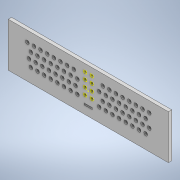
# Autodesk Inventor part: Front Panel
Saved by Autodesk Inventor 2021.4 (Build 254397000, 397)
## iProperties
Created: 2022-05-05
Part Number: Front Panel
Material: Generic
Document SubType Name: Modeling
Designer: LaborAdmin
Density: 1 g/cm^3
Appearance: Default
Author: LaborAdmin
Autodesk Inventor part; units mm, degrees
ref_plane "YZ Plane" through (0, 0, 0) normal (1, 0, 0) x (0, 1, 0)
ref_plane "XZ Plane" through (0, 0, 0) normal (0, 1, 0) x (-1, 0, 0)
ref_plane "XY Plane" through (0, 0, 0) normal (0, 0, 1) x (1, 0, 0)
sketch "Sketch1" plane through (0, 0, 0) normal (0, 0, 1) x (1, 0, 0)
  line L0 (241, -66.5) -> (-241, -66.5)
  line L1 (-241, -66.5) -> (-241, 66.5)
  line L2 (-241, 66.5) -> (241, 66.5)
  line L3 (241, 66.5) -> (241, -66.5)
  line L4 (241, -66.5) -> (-241, 66.5) construction
  line L5 (-241, -66.5) -> (241, 66.5) construction
  line L6 (197, -50) -> (-197, -50)
  line L7 (-197, -50) -> (-197, 50)
  line L8 (-197, 50) -> (197, 50)
  line L9 (197, 50) -> (197, -50)
  line L10 (197, -50) -> (-197, 50) construction
  line L11 (-197, -50) -> (197, 50) construction
  line L12 (25, 50) -> (25, -50) construction
  line L13 (-45, 50) -> (-45, -50) construction
  line L14 (-10, 45) -> (10, 45) construction
  line L15 (10, 45) -> (25, 45) construction
  line L16 (-10, 25) -> (-45, 25) construction
  line L17 (-10, 25) -> (10, 25) construction
  line L18 (-10, 5) -> (10, 5) construction
  line L19 (10, 5) -> (25, 5) construction
  arc A0 (-13.0692, 48.89) -> (-6.9308, 48.89) centre (-10, 45) ccw
  line L20 (-13.0692, 48.89) -> (-6.9308, 48.89)
  arc A1 (6.9308, 48.89) -> (13.0692, 48.89) centre (10, 45) ccw
  line L21 (6.9308, 48.89) -> (13.0692, 48.89)
  arc A2 (-13.0692, 28.89) -> (-6.9308, 28.89) centre (-10, 25) ccw
  arc A3 (6.9308, 28.89) -> (13.0692, 28.89) centre (10, 25) ccw
  arc A4 (6.9308, -11.11) -> (13.0692, -11.11) centre (10, -15) ccw
  arc A5 (-13.0692, -11.11) -> (-6.9308, -11.11) centre (-10, -15) ccw
  line L22 (-13.0692, 28.89) -> (-6.9308, 28.89)
  line L23 (6.9308, 28.89) -> (13.0692, 28.89)
  line L24 (-13.0692, -11.11) -> (-6.9308, -11.11)
  line L25 (6.9308, -11.11) -> (13.0692, -11.11)
  arc A6 (-13.0692, 8.89) -> (-6.9308, 8.89) centre (-10, 5) ccw
  arc A7 (6.9308, 8.89) -> (13.0692, 8.89) centre (10, 5) ccw
  line L26 (-13.0692, 8.89) -> (-6.9308, 8.89)
  line L27 (6.9308, 8.89) -> (13.0692, 8.89)
  line L28 (0, 0) -> (0, 31.7694) construction
  dimension "d0" = 133
  dimension "d1" = 482
  dimension "d2" = 100
  dimension "d3" = 394
  dimension "d4" = 172
  dimension "d5" = 70
  dimension "d6" = 5
  dimension "d7" = 35
  dimension "d8" = 15
  dimension "d9" = 5
  dimension "d13" = 20
  dimension "d15" = 15
  dimension "d16" = 20
  dimension "d17" = 35
  dimension "d18" = 15
  dimension "d19" = 20
  dimension "d20" = 35
  dimension "d21" = 20
  dimension "d22" = 20
  dimension "d23" = 15
  dimension "d24" = 20
  dimension "d25" = 9.91
  dimension "d26" = 3.89
  dimension "d27" = 9.91
  dimension "d28" = 3.89
  dimension "d29" = 9.91
  dimension "d30" = 9.91
  dimension "d32" = 9.91
  dimension "d33" = 35
  dimension "d34" = 9.91
  dimension "d35" = 3.89
  dimension "d36" = 3.89
  dimension "d37" = 3.89
  dimension "d38" = 3.89
  dimension "d39" = 9.91
  dimension "d40" = 9.91
  dimension "d41" = 3.89
  dimension "d42" = 3.89
  constraints: 58 end point, 16 point on circle, 10 horizontal, 8 centre point, 8 coincident, 7 perpendicular, 7 point on line, 4 midpoint, 4 parallel, 1 vertical
  measures "d0" distance of L0.end L1.end
  measures "d1" distance of L1.end L2.end
  measures "d2" distance of L6.end L7.end
  measures "d3" distance of L7.end L8.end
  measures "d4" distance of L8.end L12.start
  measures "d5" distance of L12.start L13.start
  measures "d6" distance from line of L8 L14.start
  measures "d7" distance from line of L13 L14.start
  measures "d8" distance from line of L12 L14.end
  measures "d9" distance from line of L8 L14.end
  measures "d13" distance from line of L14 L16.start
  measures "d15" distance from line of L12 L17.end
  measures "d16" distance from line of L16 L18.start
  measures "d17" distance from line of L13 L18.start
  measures "d18" distance from line of L12 L18.end
  measures "d19" distance from line of L17 L18.end
  measures "d20" distance from line of L13 L16.start
  measures "d21" distance from line of L15 L17.end
  measures "d22" distance from line of L18 point (-10, -15)
  measures "d23" distance from line of L12 point (10, -15)
  measures "d24" distance from line of L19 point (10, -15)
  measures "d25" diameter of A0
  measures "d26" distance from line of L20 A0.centre
  measures "d27" diameter of A1
  measures "d28" distance from line of L21 A1.centre
  measures "d29" diameter of A2
  measures "d30" diameter of A3
  measures "d32" diameter of A4
  measures "d33" distance from line of L13 point (-10, -15)
  measures "d34" diameter of A5
  measures "d35" distance from line of L22 L16.start
  measures "d36" distance from line of L23 L17.end
  measures "d37" distance from line of L24 point (-10, -15)
  measures "d38" distance from line of L25 point (10, -15)
  measures "d39" diameter of A6
  measures "d40" diameter of A7
  measures "d41" distance from line of L26 A6.centre
  measures "d42" distance from line of L27 L18.end
extrude "Extrusion1" add sketch "Sketch1" along normal blind 10 contours L0 L1 L2 L3 | L6 L7 L8 L9
sketch "Sketch2" plane through (0, 0, 10) normal (0, 0, 1) x (1, 0, 0)
  line L0 (6.9308, 8.89) -> (13.0692, 8.89) projected
  arc A0 (6.9308, 8.89) -> (13.0692, 8.89) centre (10, 5) ccw projected
  line L1 (-13.0692, 8.89) -> (-6.9308, 8.89) projected
  arc A1 (-13.0692, 8.89) -> (-6.9308, 8.89) centre (-10, 5) ccw projected
  line L2 (-13.0692, -11.11) -> (-6.9308, -11.11) projected
  arc A2 (-13.0692, -11.11) -> (-6.9308, -11.11) centre (-10, -15) ccw projected
  line L3 (6.9308, -11.11) -> (13.0692, -11.11) projected
  arc A3 (6.9308, -11.11) -> (13.0692, -11.11) centre (10, -15) ccw projected
  line L4 (6.9308, 28.89) -> (13.0692, 28.89) projected
  arc A4 (6.9308, 28.89) -> (13.0692, 28.89) centre (10, 25) ccw projected
  line L5 (-13.0692, 28.89) -> (-6.9308, 28.89) projected
  arc A5 (-13.0692, 28.89) -> (-6.9308, 28.89) centre (-10, 25) ccw projected
  line L6 (6.9308, 48.89) -> (13.0692, 48.89) projected
  arc A6 (6.9308, 48.89) -> (13.0692, 48.89) centre (10, 45) ccw projected
  line L7 (-13.0692, 48.89) -> (-6.9308, 48.89) projected
  arc A7 (-13.0692, 48.89) -> (-6.9308, 48.89) centre (-10, 45) ccw projected
  point P0 (0, 0)
sketch "Sketch3" plane through (0, 0, 10) normal (0, 0, 1) x (1, 0, 0)
  point P0 (0, 0)
sketch "Sketch4" plane through (0, 0, 10) normal (0, 0, 1) x (1, 0, 0)
  arc A0 (6.9308, 48.89) -> (13.0692, 48.89) centre (10, 45) ccw projected
  line L0 (9.7328, 35) -> (197, 35) construction
  line L1 (197, -50) -> (197, 50) projected
  arc A1 (6.9308, 28.89) -> (13.0692, 28.89) centre (10, 25) ccw projected
  line L2 (10, 15) -> (197, 15) construction
  arc A2 (6.9308, 8.89) -> (13.0692, 8.89) centre (10, 5) ccw projected
  line L3 (10, -5) -> (197, -5) construction
  arc A3 (6.9308, -11.11) -> (13.0692, -11.11) centre (10, -15) ccw projected
  line L4 (10, -25) -> (197, -25) construction
  line L5 (-197, -50) -> (197, -50) projected
  arc A4 (30.5999, 20.1) -> (35.2259, 20.1) centre (32.9129, 15) ccw
  arc A5 (50.5999, 20.1) -> (55.2259, 20.1) centre (52.9129, 15) ccw
  arc A6 (70.5999, 20.1) -> (75.2259, 20.1) centre (72.9129, 15) ccw
  arc A7 (90.5999, 20.1) -> (95.2259, 20.1) centre (92.9129, 15) ccw
  arc A8 (110.5999, 20.1) -> (115.2259, 20.1) centre (112.9129, 15) ccw
  arc A9 (130.5999, 20.1) -> (135.2259, 20.1) centre (132.9129, 15) ccw
  arc A10 (150.5999, 20.1) -> (155.2259, 20.1) centre (152.9129, 15) ccw
  arc A11 (170.5999, 20.1) -> (175.2259, 20.1) centre (172.9129, 15) ccw
  arc A12 (41.228, 0.1) -> (45.854, 0.1) centre (43.541, -5) ccw
  arc A13 (61.228, 0.1) -> (65.854, 0.1) centre (63.541, -5) ccw
  arc A14 (81.228, 0.1) -> (85.854, 0.1) centre (83.541, -5) ccw
  arc A15 (101.228, 0.1) -> (105.854, 0.1) centre (103.541, -5) ccw
  arc A16 (121.228, 0.1) -> (125.854, 0.1) centre (123.541, -5) ccw
  arc A17 (141.228, 0.1) -> (145.854, 0.1) centre (143.541, -5) ccw
  arc A18 (161.228, 0.1) -> (165.854, 0.1) centre (163.541, -5) ccw
  arc A19 (181.228, 0.1) -> (185.854, 0.1) centre (183.541, -5) ccw
  arc A20 (41.228, 40.1) -> (45.854, 40.1) centre (43.541, 35) ccw
  arc A21 (61.228, 40.1) -> (65.854, 40.1) centre (63.541, 35) ccw
  arc A22 (81.228, 40.1) -> (85.854, 40.1) centre (83.541, 35) ccw
  arc A23 (101.228, 40.1) -> (105.854, 40.1) centre (103.541, 35) ccw
  arc A24 (121.228, 40.1) -> (125.854, 40.1) centre (123.541, 35) ccw
  arc A25 (141.228, 40.1) -> (145.854, 40.1) centre (143.541, 35) ccw
  arc A26 (161.228, 40.1) -> (165.854, 40.1) centre (163.541, 35) ccw
  arc A27 (181.228, 40.1) -> (185.854, 40.1) centre (183.541, 35) ccw
  arc A28 (30.5999, -19.9) -> (35.2259, -19.9) centre (32.9129, -25) ccw
  arc A29 (50.5999, -19.9) -> (55.2259, -19.9) centre (52.9129, -25) ccw
  arc A30 (70.5999, -19.9) -> (75.2259, -19.9) centre (72.9129, -25) ccw
  arc A31 (90.5999, -19.9) -> (95.2259, -19.9) centre (92.9129, -25) ccw
  arc A32 (110.5999, -19.9) -> (115.2259, -19.9) centre (112.9129, -25) ccw
  arc A33 (130.5999, -19.9) -> (135.2259, -19.9) centre (132.9129, -25) ccw
  arc A34 (150.5999, -19.9) -> (155.2259, -19.9) centre (152.9129, -25) ccw
  arc A35 (170.5999, -19.9) -> (175.2259, -19.9) centre (172.9129, -25) ccw
  line L6 (181.228, 0.1) -> (185.854, 0.1)
  line L7 (161.228, 0.1) -> (165.854, 0.1)
  line L8 (141.228, 0.1) -> (145.854, 0.1)
  line L9 (121.228, 0.1) -> (125.854, 0.1)
  line L10 (101.228, 0.1) -> (105.854, 0.1)
  line L11 (81.228, 0.1) -> (85.854, 0.1)
  line L12 (41.228, 0.1) -> (45.854, 0.1)
  line L13 (61.228, 0.1) -> (65.854, 0.1)
  line L14 (41.228, 40.1) -> (45.854, 40.1)
  line L15 (61.228, 40.1) -> (65.854, 40.1)
  line L16 (81.228, 40.1) -> (85.854, 40.1)
  line L17 (101.228, 40.1) -> (105.854, 40.1)
  line L18 (121.228, 40.1) -> (125.854, 40.1)
  line L19 (141.228, 40.1) -> (145.854, 40.1)
  line L20 (161.228, 40.1) -> (165.854, 40.1)
  line L21 (181.228, 40.1) -> (185.854, 40.1)
  circle A36 centre (43.541, 35) radius 8 construction
  circle A37 centre (63.541, 35) radius 8 construction
  line L22 (30.5999, 20.1) -> (35.2259, 20.1)
  line L23 (50.5999, 20.1) -> (55.2259, 20.1)
  line L24 (70.5999, 20.1) -> (75.2259, 20.1)
  line L25 (90.5999, 20.1) -> (95.2259, 20.1)
  line L26 (110.5999, 20.1) -> (115.2259, 20.1)
  line L27 (130.5999, 20.1) -> (135.2259, 20.1)
  line L28 (150.5999, 20.1) -> (155.2259, 20.1)
  line L29 (170.5999, 20.1) -> (175.2259, 20.1)
  line L30 (30.5999, -19.9) -> (35.2259, -19.9)
  line L31 (50.5999, -19.9) -> (55.2259, -19.9)
  line L32 (70.5999, -19.9) -> (75.2259, -19.9)
  line L33 (90.5999, -19.9) -> (95.2259, -19.9)
  line L34 (110.5999, -19.9) -> (115.2259, -19.9)
  line L35 (130.5999, -19.9) -> (135.2259, -19.9)
  line L36 (150.5999, -19.9) -> (155.2259, -19.9)
  line L37 (170.5999, -19.9) -> (175.2259, -19.9)
  line L38 (6.9308, 8.89) -> (13.0692, 8.89) projected
  arc A38 (6.9308, 8.89) -> (13.0692, 8.89) centre (10, 5) ccw projected
  line L39 (-13.0692, 8.89) -> (-6.9308, 8.89) projected
  arc A39 (-13.0692, 8.89) -> (-6.9308, 8.89) centre (-10, 5) ccw projected
  line L40 (-13.0692, -11.11) -> (-6.9308, -11.11) projected
  arc A40 (-13.0692, -11.11) -> (-6.9308, -11.11) centre (-10, -15) ccw projected
  line L41 (6.9308, -11.11) -> (13.0692, -11.11) projected
  arc A41 (6.9308, -11.11) -> (13.0692, -11.11) centre (10, -15) ccw projected
  line L42 (6.9308, 28.89) -> (13.0692, 28.89) projected
  arc A42 (6.9308, 28.89) -> (13.0692, 28.89) centre (10, 25) ccw projected
  line L43 (-13.0692, 28.89) -> (-6.9308, 28.89) projected
  arc A43 (-13.0692, 28.89) -> (-6.9308, 28.89) centre (-10, 25) ccw projected
  line L44 (6.9308, 48.89) -> (13.0692, 48.89) projected
  arc A44 (6.9308, 48.89) -> (13.0692, 48.89) centre (10, 45) ccw projected
  line L45 (-13.0692, 48.89) -> (-6.9308, 48.89) projected
  arc A45 (-13.0692, 48.89) -> (-6.9308, 48.89) centre (-10, 45) ccw projected
  line L46 (241, 66.5) -> (-241, 66.5) projected
  point P0 (0, 0)
  dimension "d46" = 25
  dimension "d47" = 20
  dimension "d48" = 20
  dimension "d49" = 20
  dimension "d50" = 20
  dimension "d51" = 20
  dimension "d52" = 20
  dimension "d53" = 20
  dimension "d54" = 11.2
  dimension "d55" = 11.2
  dimension "d56" = 11.2
  dimension "d57" = 11.2
  dimension "d58" = 11.2
  dimension "d59" = 11.2
  dimension "d60" = 11.2
  dimension "d61" = 11.2
  dimension "d62" = 35
  dimension "d63" = 20
  dimension "d64" = 20
  dimension "d65" = 20
  dimension "d66" = 20
  dimension "d67" = 20
  dimension "d68" = 20
  dimension "d69" = 20
  dimension "d70" = 11.2
  dimension "d71" = 11.2
  dimension "d72" = 11.2
  dimension "d73" = 11.2
  dimension "d74" = 11.2
  dimension "d75" = 11.2
  dimension "d76" = 11.2
  dimension "d77" = 11.2
  dimension "d78" = 35
  dimension "d79" = 20
  dimension "d80" = 20
  dimension "d81" = 20
  dimension "d82" = 20
  dimension "d83" = 20
  dimension "d84" = 20
  dimension "d85" = 20
  dimension "d86" = 11.2
  dimension "d87" = 11.2
  dimension "d88" = 11.2
  dimension "d89" = 11.2
  dimension "d90" = 11.2
  dimension "d91" = 11.2
  dimension "d92" = 11.2
  dimension "d93" = 11.2
  dimension "d94" = 11.2
  dimension "d95" = 11.2
  dimension "d96" = 11.2
  dimension "d97" = 11.2
  dimension "d98" = 11.2
  dimension "d99" = 11.2
  dimension "d100" = 11.2
  dimension "d101" = 11.2
  dimension "d104" = 10.7
  dimension "d106" = 10.7
  dimension "d107" = 10.7
  dimension "d108" = 10.7
  dimension "d109" = 10.7
  dimension "d110" = 10.7
  dimension "d111" = 10.7
  dimension "d112" = 10.7
  constraints: 64 end point, 64 point on circle, 34 centre point, 34 coincident, 32 horizontal, 4 point on line, 3 vertical, 44 other
  measures "d46" distance of A1.centre point (32.913, 15)
  measures "d47" distance of point (52.913, 15) point (32.913, 15)
  measures "d48" distance of point (72.913, 15) point (52.913, 15)
  measures "d49" distance of point (92.913, 15) point (72.913, 15)
  measures "d50" distance of point (112.913, 15) point (92.913, 15)
  measures "d51" distance of point (132.913, 15) point (112.913, 15)
  measures "d52" distance of point (132.913, 15) point (152.913, 15)
  measures "d53" distance of point (172.913, 15) point (152.913, 15)
  measures "d54" diameter of A4
  measures "d55" diameter of A5
  measures "d56" diameter of A6
  measures "d57" diameter of A7
  measures "d58" diameter of A8
  measures "d59" diameter of A9
  measures "d60" diameter of A10
  measures "d61" diameter of A11
  measures "d62" distance of A2.centre point (43.541, -5)
  measures "d63" distance of point (43.541, -5) point (63.541, -5)
  measures "d64" distance of point (63.541, -5) point (83.541, -5)
  measures "d65" distance of point (83.541, -5) point (103.541, -5)
  measures "d66" distance of point (103.541, -5) point (123.541, -5)
  measures "d67" distance of point (123.541, -5) point (143.541, -5)
  measures "d68" distance of point (143.541, -5) point (163.541, -5)
  measures "d69" distance of point (163.541, -5) point (183.541, -5)
  measures "d70" diameter of A12
  measures "d71" diameter of A13
  measures "d72" diameter of A14
  measures "d73" diameter of A15
  measures "d74" diameter of A16
  measures "d75" diameter of A17
  measures "d76" diameter of A18
  measures "d77" diameter of A19
  measures "d78" distance of point (43.541, 35) A0.centre
  measures "d79" distance of point (43.541, 35) point (63.541, 35)
  measures "d80" distance of point (63.541, 35) point (83.541, 35)
  measures "d81" distance of point (83.541, 35) point (103.541, 35)
  measures "d82" distance of point (103.541, 35) point (123.541, 35)
  measures "d83" distance of point (123.541, 35) point (143.541, 35)
  measures "d84" distance of point (143.541, 35) point (163.541, 35)
  measures "d85" distance of point (163.541, 35) point (183.541, 35)
  measures "d86" diameter of A20
  measures "d87" diameter of A21
  measures "d88" diameter of A22
  measures "d89" diameter of A23
  measures "d90" diameter of A24
  measures "d91" diameter of A25
  measures "d92" diameter of A26
  measures "d93" diameter of A27
  measures "d94" diameter of A28
  measures "d95" diameter of A29
  measures "d96" diameter of A30
  measures "d97" diameter of A31
  measures "d98" diameter of A32
  measures "d99" diameter of A33
  measures "d100" diameter of A34
  measures "d101" diameter of A35
extrude "Extrusion2" cut sketch "Sketch4" against normal through all contours L22 A4 | L23 A5 | L24 A6 | L25 A7 | L26 A8 | L27 A9 | L28 A10 | L29 A11 | L12 A12 | L13 A13 | L11 A14 | L10 A15 | L9 A16 | L8 A17 | L7 A18 | L6 A19 | L14 A20 | L15 A21 | L16 A22 | L17 A23 | L18 A24 | L19 A25 | L20 A26 | L21 A27 | L30 A28 | L31 A29 | L32 A30 | L33 A31 | L34 A32 | L35 A33 | L36 A34 | L37 A35
sketch "Sketch5" plane through (0, 0, 10) normal (0, 0, 1) x (1, 0, 0)
  arc A0 (-175.2259, 20.1) -> (-170.5999, 20.1) centre (-172.9129, 15) ccw
  arc A1 (-155.2259, 20.1) -> (-150.5999, 20.1) centre (-152.9129, 15) ccw
  arc A2 (-135.2259, 20.1) -> (-130.5999, 20.1) centre (-132.9129, 15) ccw
  arc A3 (-115.2259, 20.1) -> (-110.5999, 20.1) centre (-112.9129, 15) ccw
  arc A4 (-95.2259, 20.1) -> (-90.5999, 20.1) centre (-92.9129, 15) ccw
  arc A5 (-75.2259, 20.1) -> (-70.5999, 20.1) centre (-72.9129, 15) ccw
  arc A6 (-55.2259, 20.1) -> (-50.5999, 20.1) centre (-52.9129, 15) ccw
  arc A7 (-35.2259, 20.1) -> (-30.5999, 20.1) centre (-32.9129, 15) ccw
  arc A8 (-180.5973, 0.1) -> (-175.9713, 0.1) centre (-178.2843, -5) ccw
  arc A9 (-160.5973, 0.1) -> (-155.9713, 0.1) centre (-158.2843, -5) ccw
  arc A10 (-140.5973, 0.1) -> (-135.9713, 0.1) centre (-138.2843, -5) ccw
  arc A11 (-120.5973, 0.1) -> (-115.9713, 0.1) centre (-118.2843, -5) ccw
  arc A12 (-100.5973, 0.1) -> (-95.9713, 0.1) centre (-98.2843, -5) ccw
  arc A13 (-80.5973, 0.1) -> (-75.9713, 0.1) centre (-78.2843, -5) ccw
  arc A14 (-60.5973, 0.1) -> (-55.9713, 0.1) centre (-58.2843, -5) ccw
  arc A15 (-40.5973, 0.1) -> (-35.9713, 0.1) centre (-38.2843, -5) ccw
  arc A16 (-185.854, 40.1) -> (-181.228, 40.1) centre (-183.541, 35) ccw
  arc A17 (-165.854, 40.1) -> (-161.228, 40.1) centre (-163.541, 35) ccw
  arc A18 (-145.854, 40.1) -> (-141.228, 40.1) centre (-143.541, 35) ccw
  arc A19 (-125.854, 40.1) -> (-121.228, 40.1) centre (-123.541, 35) ccw
  arc A20 (-105.854, 40.1) -> (-101.228, 40.1) centre (-103.541, 35) ccw
  arc A21 (-85.854, 40.1) -> (-81.228, 40.1) centre (-83.541, 35) ccw
  arc A22 (-65.854, 40.1) -> (-61.228, 40.1) centre (-63.541, 35) ccw
  arc A23 (-45.854, 40.1) -> (-41.228, 40.1) centre (-43.541, 35) ccw
  arc A24 (-175.2259, -19.9) -> (-170.5999, -19.9) centre (-172.9129, -25) ccw
  arc A25 (-155.2259, -19.9) -> (-150.5999, -19.9) centre (-152.9129, -25) ccw
  arc A26 (-135.2259, -19.9) -> (-130.5999, -19.9) centre (-132.9129, -25) ccw
  arc A27 (-115.2259, -19.9) -> (-110.5999, -19.9) centre (-112.9129, -25) ccw
  arc A28 (-95.2259, -19.9) -> (-90.5999, -19.9) centre (-92.9129, -25) ccw
  arc A29 (-75.2259, -19.9) -> (-70.5999, -19.9) centre (-72.9129, -25) ccw
  arc A30 (-55.2259, -19.9) -> (-50.5999, -19.9) centre (-52.9129, -25) ccw
  arc A31 (-35.2259, -19.9) -> (-30.5999, -19.9) centre (-32.9129, -25) ccw
  line L0 (-40.5973, 0.1) -> (-35.9713, 0.1)
  line L1 (-60.5973, 0.1) -> (-55.9713, 0.1)
  line L2 (-80.5973, 0.1) -> (-75.9713, 0.1)
  line L3 (-100.5973, 0.1) -> (-95.9713, 0.1)
  line L4 (-120.5973, 0.1) -> (-115.9713, 0.1)
  line L5 (-140.5973, 0.1) -> (-135.9713, 0.1)
  line L6 (-180.5973, 0.1) -> (-175.9713, 0.1)
  line L7 (-160.5973, 0.1) -> (-155.9713, 0.1)
  line L8 (-185.854, 40.1) -> (-181.228, 40.1)
  line L9 (-165.854, 40.1) -> (-161.228, 40.1)
  line L10 (-145.854, 40.1) -> (-141.228, 40.1)
  line L11 (-125.854, 40.1) -> (-121.228, 40.1)
  line L12 (-105.854, 40.1) -> (-101.228, 40.1)
  line L13 (-85.854, 40.1) -> (-81.228, 40.1)
  line L14 (-65.854, 40.1) -> (-61.228, 40.1)
  line L15 (-45.854, 40.1) -> (-41.228, 40.1)
  circle A32 centre (-183.541, 35) radius 8 construction
  circle A33 centre (-163.541, 35) radius 8 construction
  line L16 (-175.2259, 20.1) -> (-170.5999, 20.1)
  line L17 (-155.2259, 20.1) -> (-150.5999, 20.1)
  line L18 (-135.2259, 20.1) -> (-130.5999, 20.1)
  line L19 (-115.2259, 20.1) -> (-110.5999, 20.1)
  line L20 (-95.2259, 20.1) -> (-90.5999, 20.1)
  line L21 (-75.2259, 20.1) -> (-70.5999, 20.1)
  line L22 (-55.2259, 20.1) -> (-50.5999, 20.1)
  line L23 (-35.2259, 20.1) -> (-30.5999, 20.1)
  line L24 (-175.2259, -19.9) -> (-170.5999, -19.9)
  line L25 (-155.2259, -19.9) -> (-150.5999, -19.9)
  line L26 (-135.2259, -19.9) -> (-130.5999, -19.9)
  line L27 (-115.2259, -19.9) -> (-110.5999, -19.9)
  line L28 (-95.2259, -19.9) -> (-90.5999, -19.9)
  line L29 (-75.2259, -19.9) -> (-70.5999, -19.9)
  line L30 (-55.2259, -19.9) -> (-50.5999, -19.9)
  line L31 (-35.2259, -19.9) -> (-30.5999, -19.9)
  line L32 (-13.0692, 48.89) -> (-6.9308, 48.89) projected
  line L33 (41.228, 40.1) -> (45.854, 40.1) projected
  line L34 (30.5999, 20.1) -> (35.2259, 20.1) projected
  arc A34 (-13.0692, 28.89) -> (-6.9308, 28.89) centre (-10, 25) ccw projected
  arc A35 (-13.0692, 48.89) -> (-6.9308, 48.89) centre (-10, 45) ccw projected
  line L35 (41.228, 0.1) -> (45.854, 0.1) projected
  arc A36 (-13.0692, 8.89) -> (-6.9308, 8.89) centre (-10, 5) ccw projected
  line L36 (30.5999, -19.9) -> (35.2259, -19.9) projected
  arc A37 (-13.0692, -11.11) -> (-6.9308, -11.11) centre (-10, -15) ccw projected
  point P0 (0, 0)
  dimension "d151" = 20
  dimension "d152" = 20
  dimension "d153" = 20
  dimension "d154" = 20
  dimension "d155" = 20
  dimension "d156" = 20
  dimension "d157" = 20
  dimension "d158" = 11.2
  dimension "d159" = 11.2
  dimension "d160" = 11.2
  dimension "d161" = 11.2
  dimension "d162" = 11.2
  dimension "d163" = 11.2
  dimension "d164" = 11.2
  dimension "d165" = 11.2
  dimension "d166" = 20
  dimension "d167" = 20
  dimension "d168" = 20
  dimension "d169" = 20
  dimension "d170" = 20
  dimension "d171" = 20
  dimension "d172" = 20
  dimension "d173" = 11.2
  dimension "d174" = 11.2
  dimension "d175" = 11.2
  dimension "d176" = 11.2
  dimension "d177" = 11.2
  dimension "d178" = 11.2
  dimension "d179" = 11.2
  dimension "d180" = 11.2
  dimension "d181" = 20
  dimension "d182" = 20
  dimension "d183" = 20
  dimension "d184" = 20
  dimension "d185" = 20
  dimension "d186" = 20
  dimension "d187" = 20
  dimension "d188" = 11.2
  dimension "d189" = 11.2
  dimension "d190" = 11.2
  dimension "d191" = 11.2
  dimension "d192" = 11.2
  dimension "d193" = 11.2
  dimension "d194" = 11.2
  dimension "d195" = 11.2
  dimension "d196" = 11.2
  dimension "d197" = 11.2
  dimension "d198" = 11.2
  dimension "d199" = 11.2
  dimension "d200" = 11.2
  dimension "d201" = 11.2
  dimension "d202" = 11.2
  dimension "d203" = 11.2
  dimension "d204" = 10.7
  dimension "d205" = 10.7
  dimension "d206" = 10.7
  dimension "d207" = 10.7
  dimension "d208" = 10.7
  dimension "d209" = 10.7
  dimension "d210" = 10.7
  dimension "d211" = 10.7
  dimension "d212" = 10.7
  dimension "d213" = 10.7
  dimension "d214" = 20
  constraints: 64 end point, 64 point on circle, 34 centre point, 34 coincident, 32 collinear, 15 horizontal
  measures "d151" distance of point (-152.913, 15) point (-172.913, 15)
  measures "d152" distance of point (-132.913, 15) point (-152.913, 15)
  measures "d153" distance of point (-112.913, 15) point (-132.913, 15)
  measures "d154" distance of point (-92.913, 15) point (-112.913, 15)
  measures "d155" distance of point (-72.913, 15) point (-92.913, 15)
  measures "d156" distance of point (-72.913, 15) point (-52.913, 15)
  measures "d157" distance of point (-32.913, 15) point (-52.913, 15)
  measures "d158" diameter of A0
  measures "d159" diameter of A1
  measures "d160" diameter of A2
  measures "d161" diameter of A3
  measures "d162" diameter of A4
  measures "d163" diameter of A5
  measures "d164" diameter of A6
  measures "d165" diameter of A7
  measures "d166" distance of point (-178.284, -5) point (-158.284, -5)
  measures "d167" distance of point (-158.284, -5) point (-138.284, -5)
  measures "d168" distance of point (-138.284, -5) point (-118.284, -5)
  measures "d169" distance of point (-118.284, -5) point (-98.284, -5)
  measures "d170" distance of point (-98.284, -5) point (-78.284, -5)
  measures "d171" distance of point (-78.284, -5) point (-58.284, -5)
  measures "d172" distance of point (-58.284, -5) point (-38.284, -5)
  measures "d173" diameter of A8
  measures "d174" diameter of A9
  measures "d175" diameter of A10
  measures "d176" diameter of A11
  measures "d177" diameter of A12
  measures "d178" diameter of A13
  measures "d179" diameter of A14
  measures "d180" diameter of A15
  measures "d181" distance of point (-183.541, 35) point (-163.541, 35)
  measures "d182" distance of point (-163.541, 35) point (-143.541, 35)
  measures "d183" distance of point (-143.541, 35) point (-123.541, 35)
  measures "d184" distance of point (-123.541, 35) point (-103.541, 35)
  measures "d185" distance of point (-103.541, 35) point (-83.541, 35)
  measures "d186" distance of point (-83.541, 35) point (-63.541, 35)
  measures "d187" distance of point (-63.541, 35) point (-43.541, 35)
  measures "d188" diameter of A16
  measures "d189" diameter of A17
  measures "d190" diameter of A18
  measures "d191" diameter of A19
  measures "d192" diameter of A20
  measures "d193" diameter of A21
  measures "d194" diameter of A22
  measures "d195" diameter of A23
  measures "d196" diameter of A24
  measures "d197" diameter of A25
  measures "d198" diameter of A26
  measures "d199" diameter of A27
  measures "d200" diameter of A28
  measures "d201" diameter of A29
  measures "d202" diameter of A30
  measures "d203" diameter of A31
  measures "d214" distance of A24.centre point (-152.913, -25)
extrude "Extrusion3" cut sketch "Sketch5" against normal through all contours L16 A0 | L17 A1 | L18 A2 | L19 A3 | L20 A4 | L21 A5 | L22 A6 | L23 A7 | L6 A8 | L7 A9 | L5 A10 | L4 A11 | L3 A12 | L2 A13 | L1 A14 | L0 A15 | L8 A16 | L9 A17 | L10 A18 | L11 A19 | L12 A20 | L13 A21 | L14 A22 | L15 A23 | L24 A24 | L25 A25 | L26 A26 | L27 A27 | L28 A28 | L29 A29 | L30 A30 | L31 A31
sketch "Sketch6" plane through (0, 0, 10) normal (0, 0, 1) x (1, 0, 0)
  circle A0 centre (0, -40) radius 15 construction
  line L0 (-12.5, -37.5) -> (12.5, -37.5)
  line L1 (12.5, -37.5) -> (12.5, -42.5)
  line L2 (12.5, -42.5) -> (-12.5, -42.5)
  line L3 (-12.5, -42.5) -> (-12.5, -37.5)
  line L4 (-12.5, -37.5) -> (12.5, -42.5) construction
  line L5 (12.5, -37.5) -> (-12.5, -42.5) construction
  point P0 (0, 0)
  dimension "d256" = 40
  dimension "d260" = 25
  dimension "d261" = 5
  constraints: 12 end point, 2 midpoint, 2 parallel, 1 centre point, 1 horizontal, 1 perpendicular, 1 vertical alignment
  measures "d256" distance of A0.centre point (0, 0)
  measures "d260" distance of L0.start L0.end
  measures "d261" distance of L0.end L1.end
extrude "Extrusion4" cut sketch "Sketch6" against normal blind 10
body "Solid1"
